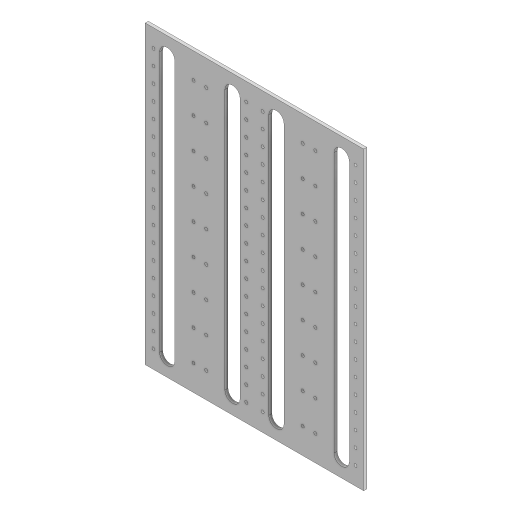
# Autodesk Inventor part: floor_ver.1
Saved by Autodesk Inventor 2024 (Build 280153000, 153)
## iProperties
Created: 2023-11-07
Part Number: floor_ver.1
Material: 一般
Document SubType Name: Modeling
Designer: bonju
Density: 1 g/cm^3
Appearance: 既定
Author: bonju
Autodesk Inventor part; units mm, degrees
ref_plane "YZ Plane" through (0, 0, 0) normal (1, 0, 0) x (0, 1, 0)
ref_plane "XZ Plane" through (0, 0, 0) normal (0, 1, 0) x (-1, 0, 0)
ref_plane "XY Plane" through (0, 0, 0) normal (0, 0, 1) x (1, 0, 0)
sketch "スケッチ1" plane through (0, 0, 0) normal (0, 0, 1) x (1, 0, 0)
  line L0 (-107, 145) -> (107, 145)
  line L1 (107, 145) -> (107, -145)
  line L2 (107, -145) -> (-107, -145)
  line L3 (-107, -145) -> (-107, 145)
  line L4 (-10817.6068, 0) -> (10817.6068, 0) projected
  line L5 (-93, -127.5) -> (-93, 127.5)
  arc A0 (-78, 127.5) -> (-93, 127.5) centre (-85.5, 127.5) ccw
  line L6 (-78, 127.5) -> (-78, -127.5)
  arc A1 (-93, -127.5) -> (-78, -127.5) centre (-85.5, -127.5) ccw
  line L7 (-29, -127.5) -> (-29, 127.5)
  arc A2 (-14, 127.5) -> (-29, 127.5) centre (-21.5, 127.5) ccw
  line L8 (-14, 127.5) -> (-14, -127.5)
  arc A3 (-29, -127.5) -> (-14, -127.5) centre (-21.5, -127.5) ccw
  line L9 (-53.5, 200.1878) -> (-53.5, -216.4934) construction
  circle A4 centre (-47.25, 120) radius 1.5
  circle A5 centre (-59.75, 120) radius 1.5
  circle A6 centre (-99, 112.5) radius 1.5
  circle A7 centre (-99, 127.5) radius 1.5
  line L10 (10710.6068, 0) -> (-10924.6068, 0)
  line L11 (0, -299.8297) -> (0, 283.524) projected
  line L12 (10817.6068, 0) -> (-10817.6068, 0)
  line L13 (53.5, 200.1878) -> (53.5, -216.4934) construction
  circle A8 centre (47.25, 120) radius 1.5
  circle A9 centre (59.75, 120) radius 1.5
  circle A10 centre (47.25, 90) radius 1.5
  circle A11 centre (59.75, 90) radius 1.5
  circle A12 centre (47.25, 60) radius 1.5
  circle A13 centre (59.75, 60) radius 1.5
  circle A14 centre (47.25, 30) radius 1.5
  circle A15 centre (59.75, 30) radius 1.5
  circle A16 centre (47.25, 0) radius 1.5
  circle A17 centre (59.75, 0) radius 1.5
  circle A18 centre (47.25, -30) radius 1.5
  circle A19 centre (59.75, -30) radius 1.5
  circle A20 centre (47.25, -60) radius 1.5
  circle A21 centre (59.75, -60) radius 1.5
  circle A22 centre (47.25, -90) radius 1.5
  circle A23 centre (59.75, -90) radius 1.5
  circle A24 centre (47.25, -120) radius 1.5
  circle A25 centre (59.75, -120) radius 1.5
  line L14 (-10710.6068, 0) -> (10924.6068, 0)
  circle A26 centre (-47.25, 90) radius 1.5
  circle A27 centre (-59.75, 90) radius 1.5
  circle A28 centre (-47.25, 60) radius 1.5
  circle A29 centre (-59.75, 60) radius 1.5
  circle A30 centre (-47.25, 30) radius 1.5
  circle A31 centre (-59.75, 30) radius 1.5
  circle A32 centre (-47.25, 0) radius 1.5
  circle A33 centre (-59.75, 0) radius 1.5
  circle A34 centre (-47.25, -30) radius 1.5
  circle A35 centre (-59.75, -30) radius 1.5
  circle A36 centre (-47.25, -60) radius 1.5
  circle A37 centre (-59.75, -60) radius 1.5
  circle A38 centre (-47.25, -90) radius 1.5
  circle A39 centre (-59.75, -90) radius 1.5
  circle A40 centre (-47.25, -120) radius 1.5
  circle A41 centre (-59.75, -120) radius 1.5
  line L15 (10817.6068, 0) -> (-10817.6068, 0)
  line L16 (93, -127.5) -> (93, 127.5)
  arc A42 (93, 127.5) -> (78, 127.5) centre (85.5, 127.5) ccw
  line L17 (78, 127.5) -> (78, -127.5)
  arc A43 (78, -127.5) -> (93, -127.5) centre (85.5, -127.5) ccw
  line L18 (29, -127.5) -> (29, 127.5)
  arc A44 (29, 127.5) -> (14, 127.5) centre (21.5, 127.5) ccw
  line L19 (14, 127.5) -> (14, -127.5)
  arc A45 (14, -127.5) -> (29, -127.5) centre (21.5, -127.5) ccw
  line L20 (-10710.6068, 0) -> (10924.6068, 0)
  line L21 (-10817.6068, 0) -> (10817.6068, 0)
  line L22 (10710.6068, 0) -> (-10924.6068, 0)
  circle A46 centre (-99, 97.5) radius 1.5
  circle A47 centre (-99, 82.5) radius 1.5
  circle A48 centre (-99, 67.5) radius 1.5
  circle A49 centre (-99, 52.5) radius 1.5
  circle A50 centre (-99, 37.5) radius 1.5
  circle A51 centre (-99, 22.5) radius 1.5
  circle A52 centre (-99, 7.5) radius 1.5
  circle A53 centre (-99, -7.5) radius 1.5
  circle A54 centre (-99, -22.5) radius 1.5
  circle A55 centre (-99, -37.5) radius 1.5
  circle A56 centre (-99, -52.5) radius 1.5
  circle A57 centre (-99, -67.5) radius 1.5
  circle A58 centre (-99, -82.5) radius 1.5
  circle A59 centre (-99, -97.5) radius 1.5
  circle A60 centre (-99, -112.5) radius 1.5
  circle A61 centre (-99, -127.5) radius 1.5
  line L23 (10710.6068, 0) -> (-10924.6068, 0)
  circle A62 centre (-8, 112.5) radius 1.5
  circle A63 centre (-8, 127.5) radius 1.5
  line L24 (-10817.6068, 0) -> (10817.6068, 0)
  line L25 (-10924.6068, 0) -> (10710.6068, 0)
  line L26 (10603.6068, 0) -> (-11031.6068, 0)
  line L27 (10603.6068, 0) -> (-11031.6068, 0)
  line L28 (-10924.6068, 0) -> (10710.6068, 0)
  line L29 (10710.6068, 0) -> (-10924.6068, 0)
  line L30 (-10817.6068, 0) -> (10817.6068, 0)
  circle A64 centre (-8, 97.5) radius 1.5
  circle A65 centre (-8, 82.5) radius 1.5
  circle A66 centre (-8, 67.5) radius 1.5
  circle A67 centre (-8, 52.5) radius 1.5
  circle A68 centre (-8, 37.5) radius 1.5
  circle A69 centre (-8, 22.5) radius 1.5
  circle A70 centre (-8, 7.5) radius 1.5
  circle A71 centre (-8, -7.5) radius 1.5
  circle A72 centre (-8, -22.5) radius 1.5
  circle A73 centre (-8, -37.5) radius 1.5
  circle A74 centre (-8, -52.5) radius 1.5
  circle A75 centre (-8, -67.5) radius 1.5
  circle A76 centre (-8, -82.5) radius 1.5
  circle A77 centre (-8, -97.5) radius 1.5
  circle A78 centre (-8, -112.5) radius 1.5
  circle A79 centre (-8, -127.5) radius 1.5
  line L31 (10817.6068, 0) -> (-10817.6068, 0)
  circle A80 centre (99, 112.5) radius 1.5
  circle A81 centre (99, 127.5) radius 1.5
  line L32 (-10710.6068, 0) -> (10924.6068, 0)
  line L33 (-10817.6068, 0) -> (10817.6068, 0)
  line L34 (10710.6068, 0) -> (-10924.6068, 0)
  line L35 (10710.6068, 0) -> (-10924.6068, 0)
  line L36 (-10817.6068, 0) -> (10817.6068, 0)
  line L37 (10817.6068, 0) -> (-10817.6068, 0)
  line L38 (-10710.6068, 0) -> (10924.6068, 0)
  circle A82 centre (99, 97.5) radius 1.5
  circle A83 centre (99, 82.5) radius 1.5
  circle A84 centre (99, 67.5) radius 1.5
  circle A85 centre (99, 52.5) radius 1.5
  circle A86 centre (99, 37.5) radius 1.5
  circle A87 centre (99, 22.5) radius 1.5
  circle A88 centre (99, 7.5) radius 1.5
  circle A89 centre (99, -7.5) radius 1.5
  circle A90 centre (99, -22.5) radius 1.5
  circle A91 centre (99, -37.5) radius 1.5
  circle A92 centre (99, -52.5) radius 1.5
  circle A93 centre (99, -67.5) radius 1.5
  circle A94 centre (99, -82.5) radius 1.5
  circle A95 centre (99, -97.5) radius 1.5
  circle A96 centre (99, -112.5) radius 1.5
  circle A97 centre (99, -127.5) radius 1.5
  circle A98 centre (8, 112.5) radius 1.5
  circle A99 centre (8, 127.5) radius 1.5
  circle A100 centre (8, -7.5) radius 1.5
  circle A101 centre (8, 97.5) radius 1.5
  circle A102 centre (8, 52.5) radius 1.5
  circle A103 centre (8, 67.5) radius 1.5
  circle A104 centre (8, 82.5) radius 1.5
  circle A105 centre (8, 37.5) radius 1.5
  circle A106 centre (8, 22.5) radius 1.5
  circle A107 centre (8, 7.5) radius 1.5
  circle A108 centre (8, -22.5) radius 1.5
  circle A109 centre (8, -37.5) radius 1.5
  circle A110 centre (8, -52.5) radius 1.5
  circle A111 centre (8, -67.5) radius 1.5
  circle A112 centre (8, -82.5) radius 1.5
  circle A113 centre (8, -97.5) radius 1.5
  circle A114 centre (8, -112.5) radius 1.5
  circle A115 centre (8, -127.5) radius 1.5
  line L39 (-10710.6068, 0) -> (10924.6068, 0)
  line L40 (10817.6068, 0) -> (-10817.6068, 0)
  line L41 (10817.6068, 0) -> (-10817.6068, 0)
  line L42 (-10603.6068, 0) -> (11031.6068, 0)
  line L43 (-10603.6068, 0) -> (11031.6068, 0)
  line L44 (10924.6068, 0) -> (-10710.6068, 0)
  line L45 (10924.6068, 0) -> (-10710.6068, 0)
  line L46 (-10710.6068, 0) -> (10924.6068, 0)
  dimension "d1" = 290
  dimension "d2" = 17.5
  dimension "d3" = 15
  dimension "d6" = 17.5
  dimension "d7" = 15
  dimension "d22" = 3
  dimension "d23" = 6.25
  dimension "d30" = 3
  dimension "d31" = 6.25
  dimension "d32" = 0
  dimension "d40" = 3
  dimension "d42" = 3
  dimension "d68" = 6
  dimension "d69" = 6
  dimension "d70" = 25
  dimension "d71" = 17.5
  dimension "d88" = 30
  dimension "d107" = 15
  dimension "d110" = 30
  constraints: 132 symmetric about line, 116 centre point, 90 end point, 16 point on circle, 8 tangent, 5 vertical, 4 parallel, 1 horizontal, 1 perpendicular, 128 other
  measures "d1" distance of L2.end L0.start
  measures "d2" distance from line of L0 A0.centre
  measures "d3" distance between parallel lines of L6 L5
  measures "d6" distance from line of L0 A2.centre
  measures "d7" distance between parallel lines of L8 L7
  measures "d22" diameter of A4
  measures "d23" distance from line of L9 A4.centre
  measures "d30" diameter of A5
  measures "d31" distance from line of L9 A5.centre
  measures "d32" vertical distance of A5.centre A4.centre
  measures "d40" diameter of A6
  measures "d42" diameter of A7
  measures "d68" distance from line of A7.centre L5
  measures "d69" distance from line of L5 A6.centre
  measures "d70" distance from line of A5.centre L0
  measures "d71" distance from line of A7.centre L0
  measures "d88" distance of A4.centre A26.centre
  measures "d107" distance of A6.centre A7.centre
  measures "d110" distance of A7.centre A46.centre
extrude "押し出し1" add sketch "スケッチ1" along normal mid plane 3 contours L0 L11 L4 L8 A2 L7 A32 A33 L6 A0 L5 L3 | L0 L1 L4 L16 A42 L17 A17 A16 L18 A44 L19 L11 | L4 L5 A1 L6 A33 A32 L7 A3 L8 L11 L2 L3 | L4 L19 A45 L18 A16 A17 L17 A43 L16 L1 L2 L11
